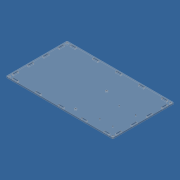
# Autodesk Inventor part: P1704_006
Saved by Autodesk Inventor 2015 SP2 (Build 190223200, 223)
## iProperties
Created: 2017-02-08
Part Number: P1704_006
Project: Manette arcade
Material: Plastique PMMA
Description: Socle
Document SubType Name: Modeling
Designer: Alexandre.PICOTTE
Authority: 315x180x4
Density: 1.188 g/cm^3
Appearance: Transparent - Clair
Mass: 263.236 g
Surface Area: 1186.04 cm^2
Volume: 221.58 cm^3
Material number: ---
Author: Boris.GAUDARD
Autodesk Inventor part; units mm, degrees
ref_plane "Plan YZ" through (0, 0, 0) normal (1, 0, 0) x (0, 1, 0)
ref_plane "Plan XZ" through (0, 0, 0) normal (0, 1, 0) x (-1, 0, 0)
ref_plane "Plan XY" through (0, 0, 0) normal (0, 0, 1) x (1, 0, 0)
sketch "Esquisse1" plane through (0, 0, 0) normal (0, 0, 1) x (1, 0, 0)
  line L0 (-157.5, 90) -> (157.5, 90)
  line L1 (157.5, 90) -> (157.5, -90)
  line L2 (157.5, -90) -> (-157.5, -90)
  line L3 (-157.5, -90) -> (-157.5, 90)
  line L4 (0, -126) -> (0, 126) construction
  line L5 (-220.5, 0) -> (220.5, 0) construction
  point P0 (0, 0)
  dimension "d0" = 315
  dimension "d1" = 180
  constraints: 8 end point, 2 parallel, 1 horizontal, 1 perpendicular, 2 other
  measures "d0" distance between parallel lines of L1 L3
  measures "d1" distance between parallel lines of L0 L2
extrude "Extrusion1" add sketch "Esquisse1" along normal blind 4
chamfer "Chanfrein1" distance 2 angle 45 4 edges at (-157.5, 90, 2) (-157.5, -90, 2) (157.5, 90, 2) (157.5, -90, 2)
sketch "Esquisse9" plane through (0, 0, 4) normal (0, 0, 1) x (1, 0, 0)
  line L0 (-142.5, 87) -> (-127.5, 87)
  line L1 (-127.5, 87) -> (-127.5, 83)
  line L2 (-127.5, 83) -> (-142.5, 83)
  line L3 (-142.5, 83) -> (-142.5, 87)
  line L4 (157.5, 90) -> (-157.5, 90) projected
  line L5 (-157.5, 90) -> (-157.5, -90) projected
  line L6 (-264.7839, 0) -> (227.8806, 0) construction
  line L7 (-75, 87) -> (-60, 87)
  line L8 (-60, 87) -> (-60, 83)
  line L9 (-60, 83) -> (-75, 83)
  line L10 (-75, 83) -> (-75, 87)
  line L11 (-7.5, 87) -> (7.5, 87)
  line L12 (7.5, 87) -> (7.5, 83)
  line L13 (7.5, 83) -> (-7.5, 83)
  line L14 (-7.5, 83) -> (-7.5, 87)
  line L15 (60, 87) -> (75, 87)
  line L16 (75, 87) -> (75, 83)
  line L17 (75, 83) -> (60, 83)
  line L18 (60, 83) -> (60, 87)
  line L19 (127.5, 87) -> (142.5, 87)
  line L20 (142.5, 87) -> (142.5, 83)
  line L21 (142.5, 83) -> (127.5, 83)
  line L22 (127.5, 83) -> (127.5, 87)
  line L23 (-142.5, -87) -> (-127.5, -87)
  line L24 (-127.5, -87) -> (-127.5, -83)
  line L25 (-127.5, -83) -> (-142.5, -83)
  line L26 (-142.5, -83) -> (-142.5, -87)
  line L27 (-75, -87) -> (-60, -87)
  line L28 (-60, -87) -> (-60, -83)
  line L29 (-60, -83) -> (-75, -83)
  line L30 (-75, -83) -> (-75, -87)
  line L31 (-7.5, -87) -> (7.5, -87)
  line L32 (7.5, -87) -> (7.5, -83)
  line L33 (7.5, -83) -> (-7.5, -83)
  line L34 (-7.5, -83) -> (-7.5, -87)
  line L35 (60, -87) -> (75, -87)
  line L36 (75, -87) -> (75, -83)
  line L37 (75, -83) -> (60, -83)
  line L38 (60, -83) -> (60, -87)
  line L39 (127.5, -87) -> (142.5, -87)
  line L40 (142.5, -87) -> (142.5, -83)
  line L41 (142.5, -83) -> (127.5, -83)
  line L42 (127.5, -83) -> (127.5, -87)
  line L43 (0, -132.9979) -> (0, 130.4487) construction
  point P0 (0, 0)
  dimension "d48" = 15
  dimension "d49" = 4
  dimension "d50" = 3
  dimension "d51" = 15
  dimension "d54" = 67.5
  constraints: 80 end point, 20 symmetric about line, 2 horizontal, 2 parallel, 1 perpendicular, 32 other
  measures "d48" distance between parallel lines of L1 L3
  measures "d49" distance between parallel lines of L0 L2
  measures "d50" distance between parallel lines of L4 L0
  measures "d51" distance between parallel lines of L3 L5
  measures "d54" distance of L0.start L7.start
extrude "Extrusion2" cut sketch "Esquisse9" against normal through all
sketch "Esquisse11" plane through (0, 0, 4) normal (0, 0, 1) x (1, 0, 0)
  line L0 (-154.5, 75) -> (-150.5, 75)
  line L1 (-150.5, 75) -> (-150.5, 60)
  line L2 (-150.5, 60) -> (-154.5, 60)
  line L3 (-154.5, 60) -> (-154.5, 75)
  line L4 (-157.5, 90) -> (-157.5, -90) projected
  line L5 (157.5, 90) -> (-157.5, 90) projected
  line L6 (0, -132.9979) -> (0, 130.4487) construction
  line L7 (-605.052, 0) -> (605.052, 0) construction
  line L8 (-154.5, 30) -> (-150.5, 30)
  line L9 (-150.5, 30) -> (-150.5, 15)
  line L10 (-150.5, 15) -> (-154.5, 15)
  line L11 (-154.5, 15) -> (-154.5, 30)
  line L12 (-154.5, -15) -> (-150.5, -15)
  line L13 (-150.5, -15) -> (-150.5, -30)
  line L14 (-150.5, -30) -> (-154.5, -30)
  line L15 (-154.5, -30) -> (-154.5, -15)
  line L16 (-154.5, -60) -> (-150.5, -60)
  line L17 (-150.5, -60) -> (-150.5, -75)
  line L18 (-150.5, -75) -> (-154.5, -75)
  line L19 (-154.5, -75) -> (-154.5, -60)
  line L20 (154.5, 75) -> (150.5, 75)
  line L21 (150.5, 75) -> (150.5, 60)
  line L22 (150.5, 60) -> (154.5, 60)
  line L23 (154.5, 60) -> (154.5, 75)
  line L24 (605.052, 0) -> (-605.052, 0) construction
  line L25 (154.5, 30) -> (150.5, 30)
  line L26 (150.5, 30) -> (150.5, 15)
  line L27 (150.5, 15) -> (154.5, 15)
  line L28 (154.5, 15) -> (154.5, 30)
  line L29 (154.5, -15) -> (150.5, -15)
  line L30 (150.5, -15) -> (150.5, -30)
  line L31 (150.5, -30) -> (154.5, -30)
  line L32 (154.5, -30) -> (154.5, -15)
  line L33 (154.5, -60) -> (150.5, -60)
  line L34 (150.5, -60) -> (150.5, -75)
  line L35 (150.5, -75) -> (154.5, -75)
  line L36 (154.5, -75) -> (154.5, -60)
  point P0 (0, 0)
  dimension "d78" = 4
  dimension "d79" = 15
  dimension "d80" = 3
  dimension "d81" = 15
  dimension "d84" = 45
  constraints: 66 end point, 18 symmetric about line, 2 parallel, 1 horizontal, 1 perpendicular, 1 vertical, 24 other
  measures "d78" distance between parallel lines of L1 L3
  measures "d79" distance between parallel lines of L2 L0
  measures "d80" distance between parallel lines of L3 L4
  measures "d81" distance between parallel lines of L5 L0
  measures "d84" distance of L0.start L8.start
extrude "Extrusion3" cut sketch "Esquisse11" against normal through all
sketch "Esquisse12" plane through (0, 0, 4) normal (0, 0, 1) x (1, 0, 0)
  point P0 (0, 0)
  point P1 (-142.5, 83)
  point P2 (-142.5, 87)
  point P3 (-127.5, 87)
  point P4 (-127.5, 83)
  point P5 (-150.5, 75)
  point P6 (-154.5, 75)
  point P7 (-154.5, 60)
  point P8 (-150.5, 60)
  point P9 (-75, 83)
  point P10 (-60, 83)
  point P11 (-60, 87)
  point P12 (-75, 87)
  point P13 (-7.5, 87)
  point P14 (-7.5, 83)
  point P15 (7.5, 87)
  point P16 (60, 87)
  point P17 (60, 83)
  point P18 (75, 83)
  point P19 (75, 87)
  point P20 (142.5, 87)
  point P21 (142.5, 83)
  point P22 (127.5, 83)
  point P23 (127.5, 87)
  point P24 (150.5, 75)
  point P25 (150.5, 60)
  point P26 (154.5, 60)
  point P27 (154.5, 30)
  point P28 (150.5, 30)
  point P29 (154.5, 15)
  point P30 (150.5, 15)
  point P31 (154.5, -60)
  point P32 (150.5, -60)
  point P33 (154.5, -30)
  point P34 (150.5, -30)
  point P35 (150.5, -15)
  point P36 (154.5, -15)
  point P37 (154.5, -75)
  point P38 (150.5, -75)
  point P39 (127.5, -87)
  point P40 (127.5, -83)
  point P41 (142.5, -83)
  point P42 (60, -87)
  point P43 (75, -87)
  point P44 (75, -83)
  point P45 (60, -83)
  point P46 (-7.5, -87)
  point P47 (-7.5, -83)
  point P48 (7.5, -83)
  point P49 (-75, -83)
  point P50 (-60, -83)
  point P51 (-60, -87)
  point P52 (-142.5, -87)
  point P53 (-127.5, -87)
  point P54 (-127.5, -83)
  point P55 (-142.5, -83)
  point P56 (-154.5, -75)
  point P57 (-154.5, -60)
  point P58 (-150.5, -60)
  point P59 (-150.5, 15)
  point P60 (-154.5, 15)
  point P61 (-150.5, -30)
  point P62 (-154.5, -30)
  point P63 (-154.5, -15)
  point P64 (-150.5, -15)
  point P65 (-150.5, 30)
  point P66 (-154.5, 30)
  point P67 (142.5, -87)
  point P68 (154.5, 75)
  point P69 (-75, -87)
  point P70 (7.5, -87)
  point P71 (-150.5, -75)
  point P72 (7.5, 83)
hole "Perçage5" at (-142.5, 83, 4) at (-142.5, 87, 4) at (-127.5, 87, 4) at (-127.5, 83, 4) at (-150.5, 75, 4) at (-154.5, 75, 4) at (-154.5, 60, 4) at (-150.5, 60, 4) at (-75, 83, 4) at (-60, 83, 4) at (-60, 87, 4) at (-75, 87, 4) at (-7.5, 87, 4) at (-7.5, 83, 4) at (7.5, 87, 4) at (60, 87, 4) at (60, 83, 4) at (75, 83, 4) at (75, 87, 4) at (142.5, 87, 4) at (142.5, 83, 4) at (127.5, 83, 4) at (127.5, 87, 4) at (150.5, 75, 4) at (150.5, 60, 4) at (154.5, 60, 4) at (154.5, 30, 4) at (150.5, 30, 4) at (154.5, 15, 4) at (150.5, 15, 4) at (154.5, -60, 4) at (150.5, -60, 4) at (154.5, -30, 4) at (150.5, -30, 4) at (150.5, -15, 4) at (154.5, -15, 4) at (154.5, -75, 4) at (150.5, -75, 4) at (127.5, -87, 4) at (127.5, -83, 4) at (142.5, -83, 4) at (60, -87, 4) at (75, -87, 4) at (75, -83, 4) at (60, -83, 4) at (-7.5, -87, 4) at (-7.5, -83, 4) at (7.5, -83, 4) at (-75, -83, 4) at (-60, -83, 4) direction (0, 0, -1) diameter 1 end through all and at (-60, -87, 4) (-142.5, -87, 4) (-127.5, -87, 4) (-127.5, -83, 4) (-142.5, -83, 4) (-154.5, -75, 4) (-154.5, -60, 4) (-150.5, -60, 4) (-150.5, 15, 4) (-154.5, 15, 4) (-150.5, -30, 4) (-154.5, -30, 4) (-154.5, -15, 4) (-150.5, -15, 4) (-150.5, 30, 4) (-154.5, 30, 4) (142.5, -87, 4) (154.5, 75, 4) (-75, -87, 4) (7.5, -87, 4) (-150.5, -75, 4) (7.5, 83, 4)
sketch "Esquisse19" plane through (0, 0, 0) normal (0, 0, -1) x (-1, 0, 0)
  line L0 (264.7839, 0) -> (-227.8806, 0) construction
  line L1 (0, -132.9979) -> (0, 130.4487) construction
  line L2 (155.5, 90) -> (-155.5, 90) construction
  line L3 (-157.5, 88) -> (-157.5, -88) construction
  point P0 (0, 0)
  point P1 (-152.5, 85)
  point P2 (152.5, 85)
  point P3 (152.5, -85)
  point P4 (-152.5, -85)
  dimension "d203" = 5
  dimension "d204" = 5
  constraints: 3 symmetric about line
  measures "d203" distance from line of L2 point (-152.5, 85)
  measures "d204" distance from line of L3 point (-152.5, 85)
hole "Perçage12" at (152.5, 85, 0) at (-152.5, 85, 0) at (-152.5, -85, 0) at (152.5, -85, 0) direction (0, 0, 1) diameter 3.4 end through all counterbore diameter 6.5 counterbore depth 2.8
sketch "Esquisse20" plane through (0, 0, 0) normal (0, 0, -1) x (-1, 0, 0)
  line L0 (-157.5, 88) -> (-157.5, -88) construction
  line L1 (-156.1923, -90) -> (154.8077, -90) construction
  line L2 (-176.0653, -60) -> (2.7327, -60) construction
  line L3 (-194.4032, 2.2) -> (-29.2901, 2.2) construction
  line L4 (-108.175, 50.3896) -> (-108.175, -85.7092) construction
  line L5 (-157.5, 88) -> (-157.5, -88) projected
  line L6 (-155.5, -90) -> (155.5, -90) projected
  point P0 (0, 0)
  point P1 (0, 0)
  point P2 (-127.5, -60)
  point P3 (-88.85, -60)
  point P4 (-132.55, 2.2)
  point P5 (-83.8, 2.2)
  dimension "d213" = 30
  dimension "d216" = 38.65
  dimension "d217" = 30
  dimension "d218" = 62.2
  dimension "d219" = 48.75
  dimension "d220" = 38.65
  constraints: 10 end point, 4 point on line, 2 collinear, 2 horizontal, 1 perpendicular, 1 symmetric about line
  measures "d213" distance between parallel lines of L1 L2
  measures "d216" distance of point (-88.85, -60) point (-127.5, -60)
  measures "d217" distance from line of L0 point (-127.5, -60)
  measures "d218" distance between parallel lines of L3 L2
  measures "d219" distance of point (-83.8, 2.2) point (-132.55, 2.2)
  measures "d220" diameter of point (-127.5, -60) L4
hole "Perçage13" at (127.5, -60, 0) at (88.85, -60, 0) at (132.55, 2.2, 0) at (83.8, 2.2, 0) direction (0, 0, 1) diameter 2.459 end through all thread size "M3x0.5" class "6H" standard "ISO M"
sketch "Esquisse14" plane through (0, 0, 4) normal (0, 0, 1) x (1, 0, 0)
  line L0 (-27.5, 92.8135) -> (-27.5, -95.3627) construction
  line L1 (-157.5, 88) -> (-157.5, -88) construction
  line L2 (-155.5, -90) -> (155.5, -90) construction
  line L3 (-176.0653, -60) -> (2.7327, -60) construction
  line L4 (-194.4032, 2.2) -> (-29.2901, 2.2) construction
  line L5 (-108.175, 50.3896) -> (-108.175, -85.7092) construction
  point P0 (0, 0)
  point P1 (-27.5, 21.5)
  point P2 (-27.5, -70)
  point P3 (-127.5, -60)
  point P4 (-88.85, -60)
  point P5 (-132.55, 2.2)
  point P6 (-83.8, 2.2)
  dimension "d128" = 130
  dimension "d136" = 30
  dimension "d137" = 20
  dimension "d138" = 91.5
  dimension "d139" = 38.65
  dimension "d140" = 30
  dimension "d141" = 62.2
  dimension "d142" = 48.75
  dimension "d143" = 38.65
  constraints: 8 end point, 6 point on line, 2 horizontal, 1 perpendicular, 1 symmetric about line, 1 vertical
  measures "d128" distance between parallel lines of L1 L0
  measures "d136" distance between parallel lines of L2 L3
  measures "d137" distance from line of L2 point (-27.5, -70)
  measures "d138" distance of point (-27.5, -70) point (-27.5, 21.5)
  measures "d139" distance of point (-88.85, -60) point (-127.5, -60)
  measures "d140" distance from line of L1 point (-127.5, -60)
  measures "d141" distance between parallel lines of L4 L3
  measures "d142" distance of point (-83.8, 2.2) point (-132.55, 2.2)
  measures "d143" diameter of point (-127.5, -60) L5
sketch "Esquisse21" plane through (0, 0, 0) normal (0, 0, -1) x (-1, 0, 0)
  line L0 (-155.5, -90) -> (155.5, -90) projected
  line L1 (-157.5, 88) -> (-157.5, -88) projected
  point P0 (0, 0)
  point P1 (0, 0)
  point P2 (-27.5, 21.5)
  point P3 (-27.5, -70)
  dimension "d231" = 91.5
  dimension "d237" = 20
  dimension "d238" = 130
  constraints: 1 vertical alignment
  measures "d231" distance of point (-27.5, -70) point (-27.5, 21.5)
  measures "d237" distance from line of L0 point (-27.5, -70)
  measures "d238" distance from line of L1 point (-27.5, -70)
hole "Perçage14" at (27.5, 21.5, 0) at (27.5, -70, 0) direction (0, 0, 1) diameter 3.4 end through all counterbore diameter 6.5 counterbore depth 2.8
equation "\"d220\" = d216"
equation "\"d143\" = d139"
